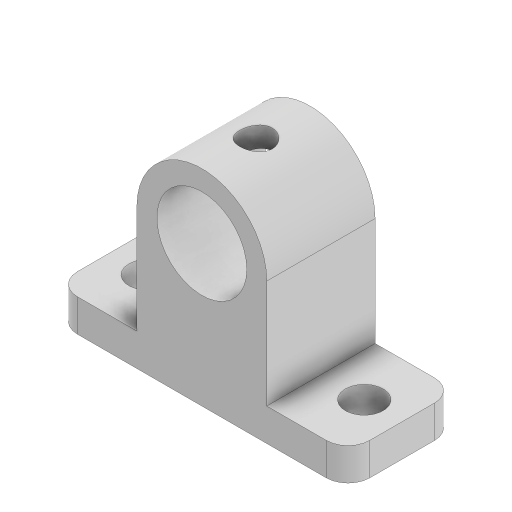
# Autodesk Inventor part: Rod Holder
Saved by Autodesk Inventor 2024 (Build 280153000, 153)
## iProperties
Created: 2025-04-26
Part Number: Rod Holder
Material: Generic
Document SubType Name: Modeling
Designer: Binara
Density: 1 g/cm^3
Appearance: Default
Author: Binara
## iProperties of the stored document Rod Holder_3DPrint.ipt
Created: 2025-04-26
Part Number: Rod Holder_3DPrint
Material: Generic
Document SubType Name: Modeling
Designer: Binara
Density: 1 g/cm^3
Appearance: Default
Author: Binara
Autodesk Inventor part; units mm, degrees
ref_plane "YZ Plane" through (0, 0, 0) normal (1, 0, 0) x (0, 1, 0)
ref_plane "XZ Plane" through (0, 0, 0) normal (0, 1, 0) x (-1, 0, 0)
sketch "Sketch1" plane through (0, 0, 0) normal (0, 0, 1) x (1, 0, 0)
  line L0 (-18.4863, -0.9573) -> (8.5137, -0.9573)
  line L1 (8.5137, -0.9573) -> (8.5137, 2.0427)
  line L2 (8.5137, 2.0427) -> (-18.4863, 2.0427)
  line L3 (-18.4863, 2.0427) -> (-18.4863, -0.9573)
  circle A0 centre (-4.9863, 12.0427) radius 4.15
  line L4 (-4.9863, 2.0427) -> (-4.9863, 12.0427)
  line L5 (-4.9863, 12.0427) -> (-4.9863, 2.0427) construction
  line L6 (-10.9863, 12.0427) -> (-10.9863, 2.0427)
  line L7 (1.0137, 2.0427) -> (1.0137, 12.0427)
  arc A1 (1.0137, 12.0427) -> (-10.9863, 12.0427) centre (-4.9863, 12.0427) ccw
  arc A2 (-10.9863, 2.0427) -> (1.0137, 2.0427) centre (-4.9863, 2.0427) ccw
  point P0 (0, 0)
  point P1 (-4.9863, 7.0427)
  point P2 (-10.9863, 2.0427)
  dimension "d0" = 3
  dimension "d1" = 27
  dimension "d2" = 8.3
  dimension "d3" = 6
  dimension "d4" = 10
  constraints: 18 end point, 4 equal length, 4 point on circle, 4 tangent, 3 centre point, 2 midpoint, 1 horizontal, 1 perpendicular, 1 vertical
  measures "d0" distance of L0.end L1.end
  measures "d1" distance of L1.end L2.end
  measures "d2" diameter of A0
  measures "d3" radius of A1
  measures "d4" distance of L4.start L4.end
extrude "Extrusion1" add sketch "Sketch1" along normal blind 10 contours L3 L2 A2 L0 | A2 L2 L0 | A2 L2 L1 L0 | L6 A1 L7 L2
sketch "Sketch2" plane through (-18.4863, -0.9573, 0) normal (0, -1, 0) x (1, 0, 0)
  line L0 (0, 0) -> (0, 10) projected
  line L1 (0, 5) -> (27, 5)
  line L2 (27, 0) -> (27, 10) projected
  circle A0 centre (3.5, 5) radius 1.75
  line L3 (19.5, 0) -> (7.5, 0) projected
  line L4 (13.5, 0) -> (13.5, -6.2833)
  circle A1 centre (23.5, 5) radius 1.75
  point P0 (18.4863, 0)
  dimension "d7" = 3.5
  dimension "d8" = 20
  constraints: 4 end point, 3 midpoint, 2 centre point, 1 point on line, 1 symmetric about line, 1 vertical, 1 other
  measures "d7" diameter of A0
  measures "d8" distance of A1.centre A0.centre
extrude "Extrusion2" cut sketch "Sketch2" against normal up to surface (3 mm away)
fillet "Fillet1" radius 2 4 edges at (-18.4863, 0.5427, 0) (-18.4863, 0.5427, 10) (8.5137, 0.5427, 0) (8.5137, 0.5427, 10)
ref_plane "Work Plane1" through (1.0137, 23.2927, 10) normal (0, 1, 0) x (1, 0, 0)
sketch "Sketch3" plane through (1.0137, 23.2927, 10) normal (0, 1, 0) x (1, 0, 0)
  line L0 (0, 10) -> (-12, 10) projected
  line L1 (-12, 10) -> (-12, 0) projected
  line L2 (0, 0) -> (-12, 0) projected
  line L3 (0, 10) -> (0, 0) projected
  line L4 (-6, 10) -> (-6, 0)
  circle A0 centre (-6, 5) radius 1.5
  point P0 (-1.0137, 10)
  dimension "d13" = 3
  constraints: 3 midpoint, 2 end point, 1 centre point
  measures "d13" diameter of A0
extrude "Extrusion3" cut sketch "Sketch3" against normal blind 10 contours A0 L4 | L4 A0
body "Solid1"
